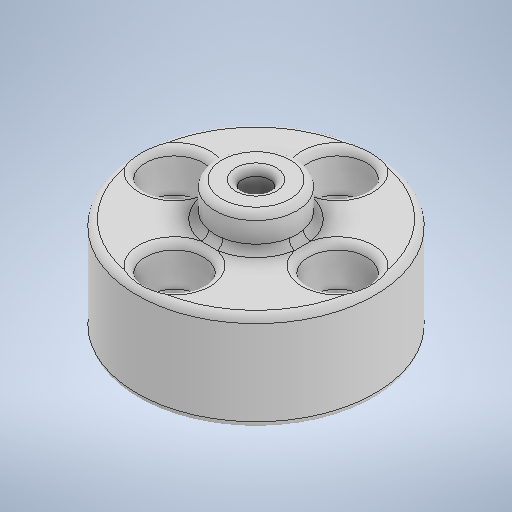
# Autodesk Inventor part: Pièce1
Saved by Autodesk Inventor 2025.1 (Build 291241000, 241)
## iProperties
Created: 2025-05-14
Part Number: Pièce1
Material: Générique
Document SubType Name: Modeling
Designer: chapuzet
Density: 1 g/cm^3
Appearance: Par défaut
Author: chapuzet
Autodesk Inventor part; units mm, degrees
ref_plane "YZ Plane" through (0, 0, 0) normal (1, 0, 0) x (0, 1, 0)
ref_plane "XZ Plane" through (0, 0, 0) normal (0, 1, 0) x (-1, 0, 0)
ref_plane "XY Plane" through (0, 0, 0) normal (0, 0, 1) x (1, 0, 0)
sketch "Esquisse1" plane through (0, 0, 0) normal (0, 1, 0) x (-1, 0, 0)
  circle A0 centre (0, 0) radius 17.5
  circle A1 centre (0, 0) radius 12
  circle A2 centre (0, -12) radius 2
  circle A3 centre (12, 0) radius 2
  circle A4 centre (0, 12) radius 2
  circle A5 centre (-12, 0) radius 2
  dimension "d1" = 24
  dimension "d0" = 35
  dimension "d2" = 4
  dimension "d11" = 360
  constraints: 5 centre point, 2 coincident, 1 vertical alignment, 11 other
  measures "d0" diameter of A0
  measures "d2" diameter of A2
extrude "Extrusion1" add sketch "Esquisse1" along normal blind 14.5 contours A0 | A3 A1 A2 A5 A4
sketch "Esquisse2" plane through (0, 14.5, 0) normal (0, 1, 0) x (1, 0, 0)
  circle A0 centre (0, 12) radius 2 projected
  circle A1 centre (0, 12) radius 4.25
  circle A2 centre (-12, 0) radius 4.25
  circle A3 centre (0, -12) radius 4.25
  circle A4 centre (12, 0) radius 4.25
  point P0 (0, 0)
  dimension "d13" = 8.5
  dimension "d16" = 360
  constraints: 4 centre point, 1 coincident, 9 other
  measures "d13" diameter of A1
extrude "Extrusion2" cut sketch "Esquisse2" against normal blind 6
sketch "Esquisse6" plane through (0, 0, 0) normal (0, -1, 0) x (1, 0, 0)
  circle A0 centre (0, 0) radius 5
  line L0 (3.75, -3.75) -> (-3.0455, 3.0455) construction
  line L1 (-3.75, 3.75) -> (3.75, 3.75)
  line L2 (3.75, 3.75) -> (3.75, -3.75)
  line L3 (3.75, -3.75) -> (-3.75, -3.75)
  line L4 (-3.75, -3.75) -> (-3.75, 3.75)
  line L5 (-3.75, 3.75) -> (3.75, -3.75) construction
  line L6 (3.75, 3.75) -> (-3.75, -3.75) construction
  line L7 (1.3726, 5.1226) -> (5.1226, -1.3726)
  line L8 (-5.1226, 1.3726) -> (1.3726, 5.1226)
  line L9 (-1.3726, -5.1226) -> (-5.1226, 1.3726)
  line L10 (5.1226, -1.3726) -> (-1.3726, -5.1226)
  line L11 (-5.1226, -1.3726) -> (-1.3726, 5.1226)
  line L12 (1.3726, -5.1226) -> (-5.1226, -1.3726)
  line L13 (5.1226, 1.3726) -> (1.3726, -5.1226)
  line L14 (-1.3726, 5.1226) -> (5.1226, 1.3726)
  point P0 (2.1651, -3.75)
  point P1 (4.3301, 0)
  point P2 (2.1651, 3.75)
  point P3 (-2.1651, 3.75)
  point P4 (-4.3301, 0)
  point P5 (-2.1651, -3.75)
  dimension "d33" = 10
  dimension "d43" = 7.5
  dimension "d46" = 360
  dimension "d48" = 7.5
  constraints: 30 end point, 2 coincident, 2 midpoint, 2 parallel, 1 centre point, 1 horizontal, 1 perpendicular, 1 point on line, 25 other
  measures "d33" diameter of A0
  measures "d43" distance of L0.start L3.end
  measures "d48" distance of L1.end L0.start
extrude "Extrusion4" cut sketch "Esquisse6" against normal blind 5.5 contours L13 L2 L7 | L2 L13 L10 L3 L12 L9 L4 L11 L8 L1 L14 L7 | L14 L1 L7 | L13 L3 L10 | L8 L11 L1 | L3 L9 L12 | L4 L9 L11
sketch "Esquisse3" plane through (0, 14.5, 0) normal (0, 1, 0) x (1, 0, 0)
  circle A0 centre (0, 0) radius 6
  dimension "d20" = 12
  constraints: 1 centre point, 1 coincident
  measures "d20" diameter of A0
extrude "Extrusion3" add sketch "Esquisse3" along normal blind 5
sketch "Esquisse5" plane through (0, 0, 0) normal (0, -1, 0) x (1, 0, 0)
  circle A0 centre (0, 0) radius 1.5
  dimension "d24" = 3
  constraints: 1 centre point, 1 coincident
  measures "d24" diameter of A0
hole "Perçage1" at (0, 0, 0) direction (0, 1, 0) diameter 4 end through all
fillet "Congé2" radius 1 13 edges at (17.5, 0, 0) (14, 0, 0) (2, 0, -12) (-10, 0, 0) (2, 0, 12) (17.5, 14.5, 0) (7.75, 14.5, 0) (-4.25, 14.5, -12) (-16.25, 14.5, 0) (-4.25, 14.5, 12) (-6, 14.5, 0) (0, 19.5, 2) (-6, 19.5, 0)
